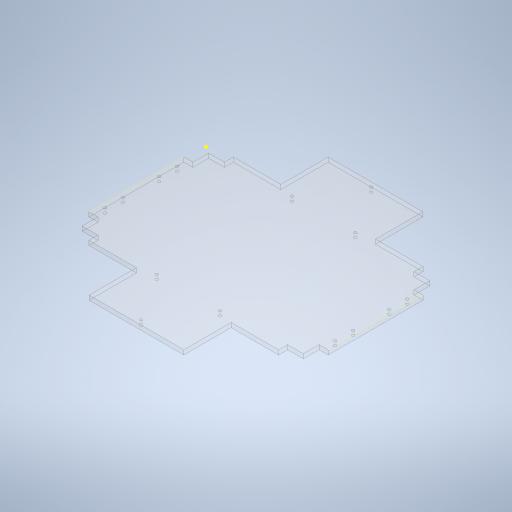
# Autodesk Inventor part: Polyc_for_swerve
Saved by Autodesk Inventor 2024 (Build 280153000, 153)
## iProperties
Created: 2023-10-23
Part Number: Polyc_for_swerve
Material: Polycarbonate, Clear
Document SubType Name: Modeling
Designer: s137416
Density: 1.2 g/cm^3
Appearance: Polycarbonate - Clear
Author: s137416
Autodesk Inventor part; units mm, degrees
ref_plane "YZ Plane" through (0, 0, 0) normal (1, 0, 0) x (0, 1, 0)
ref_plane "XZ Plane" through (0, 0, 0) normal (0, 1, 0) x (-1, 0, 0)
ref_plane "XY Plane" through (0, 0, 0) normal (0, 0, 1) x (1, 0, 0)
sketch "Sketch1" plane through (0, 0, 0) normal (0, 1, 0) x (-1, 0, 0)
  line L0 (-666.6265, 392.3922) -> (-666.6265, -14.0078)
  line L1 (6.4735, -14.0078) -> (6.4735, 392.3922)
  line L2 (-196.7265, 392.3922) -> (-196.7265, 525.7422)
  line L3 (-196.7265, 525.7422) -> (-463.4265, 525.7422)
  line L4 (-463.4265, 525.7422) -> (-463.4265, 392.3922)
  line L5 (6.4735, 392.3922) -> (-196.7265, 392.3922)
  line L6 (-463.4265, 392.3922) -> (-666.6265, 392.3922)
  line L7 (-196.7265, -14.0078) -> (-196.7265, -147.3578)
  line L8 (-196.7265, -147.3578) -> (-463.4265, -147.3578)
  line L9 (-463.4265, -147.3578) -> (-463.4265, -14.0078)
  line L10 (-666.6265, -14.0078) -> (-463.4265, -14.0078)
  line L11 (-196.7265, -14.0078) -> (6.4735, -14.0078)
  point P0 (0, 0)
  dimension "d0" = 673.1
  dimension "d1" = 406.4
  dimension "d73" = 266.7
  dimension "d75" = 203.2
  dimension "d76" = 266.7
  constraints: 24 end point, 7 parallel, 2 horizontal, 2 perpendicular
  measures "d0" distance of L1.start L0.end
  measures "d1" distance of L1.start L1.end
  measures "d73" distance of L3.end L2.end
  measures "d75" distance between parallel lines of L0 L4
  measures "d76" distance of L7.end L8.end
extrude "Extrusion1" add sketch "Sketch1" along normal blind 12.7
sketch "Sketch2" plane through (0, 12.7, 0) normal (0, 1, 0) x (1, 0, 0)
  line L0 (666.6265, -392.3922) -> (666.6265, 14.0078) projected
  line L1 (666.6265, -392.3922) -> (666.6265, -290.7922)
  line L2 (666.6265, -290.7922) -> (666.6265, -189.1922) construction
  line L3 (666.6265, 14.0078) -> (666.6265, -58.7236) construction
  line L4 (666.6265, 14.0078) -> (666.6265, -87.5922) construction
  line L5 (-6.4735, 14.0078) -> (-6.4735, -392.3922) construction
  line L6 (-6.4735, -392.3922) -> (241.1765, -392.3922) construction
  line L7 (-6.4735, -392.3922) -> (666.6265, -392.3922) construction
  line L8 (666.6265, -392.3922) -> (418.9765, -392.3922) construction
  circle A0 centre (653.9265, -290.7922) radius 3.175
  circle A1 centre (653.9265, -87.5922) radius 3.175
  circle A2 centre (241.1765, -379.6922) radius 3.175
  circle A3 centre (418.9765, -379.6922) radius 3.175
  circle A4 centre (418.9765, 1.3078) radius 3.175
  circle A5 centre (241.1765, 1.3078) radius 3.175
  circle A6 centre (6.2265, -87.5922) radius 3.175
  circle A7 centre (6.2265, -290.7922) radius 3.175
  circle A8 centre (6.2265, -239.9922) radius 3.9751
  circle A9 centre (6.2265, -138.3922) radius 3.9751
  circle A10 centre (653.9265, -239.9922) radius 3.9751
  circle A11 centre (653.9265, -138.3922) radius 3.9751
  line L9 (458.3979, 14.0078) -> (460.8865, 14.0078)
  line L10 (460.8865, 14.0078) -> (460.8865, -3.7722)
  line L11 (460.8865, -3.7722) -> (448.1865, -3.7722)
  line L12 (448.1865, -3.7722) -> (448.1865, 7.197)
  line L13 (448.1865, 7.197) -> (460.8865, 7.197)
  line L14 (460.8865, 7.197) -> (460.8865, -3.7722)
  line L15 (666.6265, 14.0078) -> (-6.4735, 14.0078) projected
  circle A12 centre (330.0765, -513.0422) radius 3.9751
  line L16 (196.7265, -392.3922) -> (196.7265, -525.7422) projected
  circle A13 centre (330.0765, 134.6578) radius 3.9751
  line L17 (196.7265, 147.3578) -> (196.7265, 14.0078) projected
  line L18 (196.7265, -525.7422) -> (463.4265, -525.7422) projected
  line L19 (463.4265, 147.3578) -> (196.7265, 147.3578) projected
  point P0 (0, 0)
  dimension "d11" = 6.35
  dimension "d12" = 6.35
  dimension "d13" = 12.7
  dimension "d14" = 12.7
  dimension "d15" = 6.35
  dimension "d16" = 12.7
  dimension "d17" = 6.35
  dimension "d18" = 12.7
  dimension "d19" = 6.35
  dimension "d20" = 6.35
  dimension "d23" = 6.35
  dimension "d24" = 6.35
  dimension "d25" = 12.7
  dimension "d26" = 12.7
  dimension "d34" = 7.9502
  dimension "d35" = 7.9502
  dimension "d40" = 50.8
  dimension "d43" = 50.8
  dimension "d44" = 7.9502
  dimension "d45" = 7.9502
  dimension "d46" = 50.8
  dimension "d66" = 205.74
  dimension "d68" = 12.7
  dimension "d70" = 17.78
  dimension "d78" = 7.9502
  dimension "d79" = 133.35
  dimension "d80" = 7.9502
  dimension "d81" = 133.35
  dimension "d82" = 12.7
  dimension "d83" = 12.7
  constraints: 24 end point, 14 centre point, 5 point on line, 2 horizontal, 2 parallel, 2 perpendicular, 1 midpoint
  measures "d11" diameter of A0
  measures "d12" diameter of A1
  measures "d13" distance from line of L0 A0.centre
  measures "d14" distance from line of L0 A1.centre
  measures "d15" diameter of A2
  measures "d16" distance from line of L7 A2.centre
  measures "d17" diameter of A3
  measures "d18" distance from line of L7 A3.centre
  measures "d19" diameter of A4
  measures "d20" diameter of A5
  measures "d23" diameter of A6
  measures "d24" diameter of A7
  measures "d25" distance from line of L5 A6.centre
  measures "d26" distance from line of L5 A7.centre
  measures "d34" diameter of A8
  measures "d35" diameter of A9
  measures "d40" distance of A9.centre A6.centre
  measures "d43" distance of A8.centre A7.centre
  measures "d44" diameter of A10
  measures "d45" diameter of A11
  measures "d46" distance of A0.centre A10.centre
  measures "d66" distance between parallel lines of L0 L10
  measures "d68" distance of L12.end L13.end
  measures "d70" distance between parallel lines of L15 L11
  measures "d78" diameter of A12
  measures "d79" distance from line of A12.centre L16
  measures "d80" diameter of A13
  measures "d81" distance from line of L17 A13.centre
  measures "d82" distance from line of L18 A12.centre
  measures "d83" distance from line of L19 A13.centre
hole "Hole1" at (653.9265, 12.7, 290.7922) at (653.9265, 12.7, 87.5922) at (418.9765, 12.7, -1.3078) at (241.1765, 12.7, -1.3078) at (418.9765, 12.7, 379.6922) at (241.1765, 12.7, 379.6922) at (6.2265, 12.7, 290.7922) at (6.2265, 12.7, 87.5922) at (6.2265, 12.7, 239.9922) at (6.2265, 12.7, 138.3922) at (653.9265, 12.7, 239.9922) at (653.9265, 12.7, 138.3922) at (330.0765, 12.7, 513.0422) at (330.0765, 12.7, -134.6578) direction (0, -1, 0) diameter 7.9502 end through all
sketch "Sketch3" plane through (0, 12.7, 0) normal (0, 1, 0) x (1, 0, 0)
  line L0 (-6.4735, -392.3922) -> (666.6265, -392.3922) projected
  line L1 (-6.4735, -392.3922) -> (63.1225, -392.3922)
  line L2 (63.1225, -392.3922) -> (63.1225, -366.9922)
  line L3 (63.1225, -366.9922) -> (18.9265, -366.9922)
  line L4 (-6.4735, -366.9922) -> (-6.4735, -392.3922)
  line L5 (-6.4735, -392.3922) -> (18.9265, -392.3922)
  line L6 (18.9265, -366.9922) -> (18.9265, -322.7962)
  line L7 (18.9265, -322.7962) -> (-6.4735, -322.7962)
  line L8 (-6.4735, -322.7962) -> (-6.4735, -392.3922)
  line L9 (666.6265, 14.0078) -> (-6.4735, 14.0078) projected
  line L10 (-6.4735, 14.0078) -> (63.1225, 14.0078)
  line L11 (63.1225, 14.0078) -> (63.1225, -11.3922)
  line L12 (63.1225, -11.3922) -> (18.9265, -11.3922)
  line L13 (-6.4735, -11.3922) -> (-6.4735, 14.0078)
  line L14 (-6.4735, 14.0078) -> (18.9265, 14.0078)
  line L15 (18.9265, -11.3922) -> (18.9265, -55.5882)
  line L16 (18.9265, -55.5882) -> (-6.4735, -55.5882)
  line L17 (-6.4735, -55.5882) -> (-6.4735, 14.0078)
  line L18 (666.6265, -392.3922) -> (641.2265, -392.3922)
  line L19 (641.2265, -366.9922) -> (641.2265, -322.7962)
  line L20 (641.2265, -322.7962) -> (666.6265, -322.7962)
  line L21 (666.6265, -322.7962) -> (666.6265, -392.3922)
  line L22 (666.6265, -392.3922) -> (597.0305, -392.3922)
  line L23 (597.0305, -392.3922) -> (597.0305, -366.9922)
  line L24 (597.0305, -366.9922) -> (641.2265, -366.9922)
  line L25 (666.6265, -366.9922) -> (666.6265, -392.3922)
  line L26 (666.6265, 14.0078) -> (597.0305, 14.0078)
  line L27 (597.0305, 14.0078) -> (597.0305, -11.3922)
  line L28 (597.0305, -11.3922) -> (641.2265, -11.3922)
  line L29 (666.6265, -11.3922) -> (666.6265, 14.0078)
  line L30 (666.6265, 14.0078) -> (641.2265, 14.0078)
  line L31 (641.2265, -11.3922) -> (641.2265, -55.5882)
  line L32 (641.2265, -55.5882) -> (666.6265, -55.5882)
  line L33 (666.6265, -55.5882) -> (666.6265, 14.0078)
  point P0 (0, 0)
  dimension "d47" = 69.596
  dimension "d48" = 25.4
  dimension "d49" = 25.4
  dimension "d50" = 69.596
  dimension "d51" = 69.596
  dimension "d52" = 25.4
  dimension "d53" = 25.4
  dimension "d54" = 69.596
  dimension "d55" = 25.4
  dimension "d56" = 69.596
  dimension "d57" = 69.596
  dimension "d58" = 25.4
  dimension "d59" = 69.596
  dimension "d60" = 25.4
  dimension "d61" = 25.4
  dimension "d62" = 69.596
  constraints: 64 end point, 16 parallel, 8 horizontal, 8 perpendicular
  measures "d47" distance of L4.start L2.end
  measures "d48" distance of L1.end L2.end
  measures "d49" distance of L7.end L6.end
  measures "d50" distance of L5.end L6.end
  measures "d51" distance of L11.end L13.start
  measures "d52" distance of L10.end L11.end
  measures "d53" distance of L15.end L16.end
  measures "d54" distance of L14.end L15.end
  measures "d55" distance of L19.end L20.end
  measures "d56" distance of L18.end L19.end
  measures "d57" distance of L23.end L25.start
  measures "d58" distance of L22.end L23.end
  measures "d59" distance of L29.start L27.end
  measures "d60" distance of L26.end L27.end
  measures "d61" distance of L32.end L31.end
  measures "d62" distance of L30.end L31.end
extrude "Extrusion2" cut sketch "Sketch3" against normal blind 25.4
sketch "Sketch4" plane through (0, 12.7, 0) normal (0, 1, 0) x (1, 0, 0)
  line L0 (-6.4735, -55.5882) -> (-6.4735, -322.7962) construction
  line L1 (666.6265, -322.7962) -> (666.6265, -55.5882) construction
  point P0 (0, 0)
body "Solid1"
